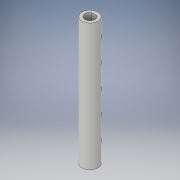
# Autodesk Inventor part: SpinnerV6
Saved by Autodesk Inventor 2019 (Build 230136000, 136)
## iProperties
Created: 2018-11-08
Part Number: SpinnerV6
Material: Generic
Document SubType Name: Modeling
Designer: Ashley
Density: 1 g/cm^3
Appearance: Default
Author: Ashley
Autodesk Inventor part; units mm, degrees
ref_plane "YZ Plane" through (0, 0, 0) normal (1, 0, 0) x (0, 1, 0)
ref_plane "XZ Plane" through (0, 0, 0) normal (0, 1, 0) x (-1, 0, 0)
ref_plane "XY Plane" through (0, 0, 0) normal (0, 0, 1) x (1, 0, 0)
sketch "Shaft Sketch" plane through (0, 0, 0) normal (0, 1, 0) x (-1, 0, 0)
  circle A0 centre (0, 0.05) radius 6
  circle A1 centre (0, 0.05) radius 6
  arc A2 (1.9691, -3.2) -> (-1.9691, -3.2) centre (0, 0.05) ccw
  line L0 (1.9691, -3.2) -> (-1.9691, -3.2)
  point P0 (0, 3.0022)
  dimension "d0" = 12
  dimension "d1" = 7.6
  dimension "d3" = 3.25
  constraints: 3 centre point, 2 coincident, 2 end point, 2 point on circle, 1 horizontal, 1 other
  measures "d0" diameter of A0
  measures "d1" diameter of A2
  measures "d3" distance from line of point (0, 0.05) L0
extrude "Shaft Extrusion" add sketch "Shaft Sketch" along normal blind 96
ref_plane "Tangent" through (0, 0, -5.95) normal (0, 0, 1) x (1, 0, 0)
sketch "Holes Sketch" plane through (0, 0, -5.95) normal (0, 0, 1) x (1, 0, 0)
  line L0 (0, 109.8875) -> (0, -25.05) construction
  line L1 (44.45, 48) -> (-58.7375, 48) construction
  line L2 (6, 96) -> (-6, 96) projected
  line L3 (-6, 0) -> (6, 0) projected
  circle A0 centre (0, 48) radius 3.75
  circle A1 centre (0, 31) radius 3.75
  circle A2 centre (0, 65) radius 3.75
  circle A3 centre (0, 48) radius 3.75
  circle A4 centre (0, 82) radius 3.75
  circle A5 centre (0, 65) radius 3.75
  circle A6 centre (0, 14) radius 3.75
  circle A7 centre (0, 31) radius 3.75
  circle A8 centre (0, 48) radius 3.75
  point P0 (0, 0)
  dimension "d6" = 48
  dimension "d9" = 7.5
  dimension "d12" = 17
  dimension "d15" = 17
  dimension "d20" = 14
  dimension "d21" = 31
  dimension "d25" = 17
  dimension "d26" = 96
  dimension "d28" = 48
  dimension "d29" = 14
  constraints: 9 centre point, 4 end point, 3 vertical, 2 point on line, 1 horizontal, 16 other
  measures "d6" distance between parallel lines of L1 L2
  measures "d9" diameter of A0
  measures "d12" distance of A0.centre A1.centre
  measures "d15" distance of A0.centre A2.centre
  measures "d20" distance from line of A4.centre L2
  measures "d21" distance from line of L3 A1.centre
  measures "d25" distance from line of L1 A2.centre
  measures "d26" distance between parallel lines of L3 L2
  measures "d28" distance between parallel lines of L3 L1
  measures "d29" distance from line of L3 A6.centre
extrude "Extrusion3" cut sketch "Holes Sketch" along normal up to next
body "Solid1"
